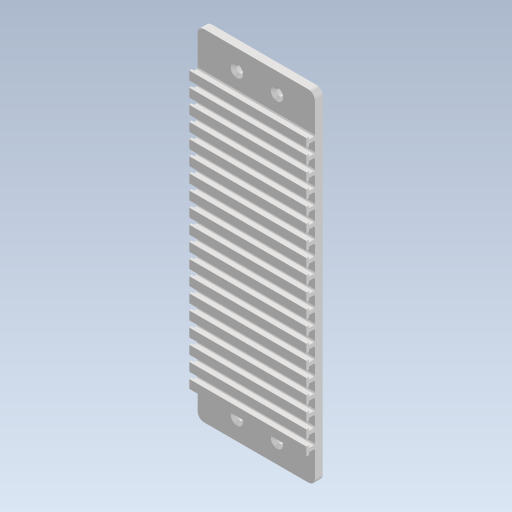
# Autodesk Inventor part: picadilly
Saved by Autodesk Inventor 2024 (Build 280153000, 153)
## iProperties
Created: 2024-06-10
Part Number: picadilly
Material: Типовые
Document SubType Name: Modeling
Designer: zhmis
Density: 1 g/cm^3
Appearance: По умолчанию
Author: zhmis
Autodesk Inventor part; units mm, degrees
ref_plane "YZ Plane" through (0, 0, 0) normal (1, 0, 0) x (0, 1, 0)
ref_plane "XZ Plane" through (0, 0, 0) normal (0, 1, 0) x (-1, 0, 0)
ref_plane "XY Plane" through (0, 0, 0) normal (0, 0, 1) x (1, 0, 0)
ref_plane "РабПлоскость1" through (0, 0, 0) normal (0, 0, 1) x (1, 0, 0)
sketch "Эскиз1" plane through (0, 0, 0) normal (0, 0, 1) x (1, 0, 0)
  circle A0 centre (-33.1299, -115.05) radius 1.65 projected
  circle A1 centre (-12.8537, -115.05) radius 1.65 projected
  circle A2 centre (-33.1299, 37.05) radius 1.65 projected
  circle A3 centre (-12.8537, 37.05) radius 1.65 projected
  line L0 (-52.9918, -117.55) -> (-52.9918, -99.275) projected
  line L1 (2.5082, -125.05) -> (-48.4918, -125.05) projected
  line L2 (2.5082, 47.05) -> (-48.4918, 47.05) projected
  line L3 (-52.9918, 39.55) -> (-52.9918, 21.275) projected
  line L4 (-52.9918, 43.875) -> (-52.9918, -121.875)
  line L5 (-49.8168, -125.05) -> (3.1042, -125.05)
  line L6 (6.2792, -121.875) -> (6.2792, 43.875)
  line L7 (3.1042, 47.05) -> (-49.8168, 47.05)
  arc A4 (-49.8168, 47.05) -> (-52.9918, 43.875) centre (-49.8168, 43.875) ccw
  arc A5 (6.2792, 43.875) -> (3.1042, 47.05) centre (3.1042, 43.875) ccw
  arc A6 (3.1042, -125.05) -> (6.2792, -121.875) centre (3.1042, -121.875) ccw
  arc A7 (-52.9918, -121.875) -> (-49.8168, -125.05) centre (-49.8168, -121.875) ccw
  point P0 (0, 0)
  point P1 (6.2792, 30.05)
  point P2 (-52.9918, 47.05)
  point P3 (-52.9918, -125.05)
  dimension "d0" = 3.175
  constraints: 8 end point, 8 point on circle, 8 tangent, 6 point on line, 4 centre point, 3 equal radius, 2 parallel, 1 perpendicular, 1 other
  measures "d0" radius of A4
extrude "Выдавливание1" add sketch "Эскиз1" along normal blind 4 contours A0 | A1 | A2 | A3 | L0 L4 L3 A4 L7 L2 A5 L6 A6 L5 L1 A7
sketch "Эскиз2" plane through (0, 0, 4) normal (0, 0, 1) x (1, 0, 0)
  circle A0 centre (-33.1299, -115.05) radius 1.65 projected
  circle A1 centre (-12.8537, -115.05) radius 1.65 projected
  circle A2 centre (-33.1299, 37.05) radius 1.65 projected
  circle A3 centre (-12.8537, 37.05) radius 1.65 projected
  point P0 (0, 0)
hole "Отверстие1" at (-12.8537, 37.05, 4) at (-33.1299, 37.05, 4) at (-12.8537, -115.05, 4) at (-33.1299, -115.05, 4) direction (0, 0, -1) diameter 3.4 depth 8.8 tip angle 118 countersink diameter 6.3 countersink angle 90 clearance for "Винт с потайной головкой ISO 2009/7046" size "M3" standard "ISO"
sketch "Эскиз4" plane through (-52.9918, -121.875, 0) normal (-1, 0, 0) x (0, 0, 1)
  line L0 (6.9999, 154.5045) -> (8.2499, 154.5045)
  line L1 (8.2499, 154.5045) -> (8.2499, 158.8045)
  line L2 (8.2499, 158.8045) -> (6.9999, 158.8045)
  line L3 (6.9999, 158.8045) -> (6.9999, 157.6045)
  line L4 (6.9999, 157.6045) -> (4.4999, 157.6045)
  line L5 (4.4999, 157.6045) -> (4.2499, 157.8545)
  line L6 (4.2499, 155.4545) -> (4.4999, 155.7045)
  line L7 (4.4999, 155.7045) -> (6.9999, 155.7045)
  line L8 (6.9999, 155.7045) -> (6.9999, 154.5045)
  line L9 (4.2499, 155.4545) -> (4, 155.2045)
  line L10 (4, 158.1044) -> (4.2499, 157.8545)
  line L11 (4, 158.1044) -> (4, 155.2045)
  line L12 (6.9999, 151.3045) -> (6.9999, 150.1045)
  line L13 (4.2499, 147.9545) -> (4, 147.7045)
  line L14 (4.4999, 150.1045) -> (4.2499, 150.3545)
  line L15 (4, 150.6044) -> (4.2499, 150.3545)
  line L16 (6.9999, 150.1045) -> (4.4999, 150.1045)
  line L17 (8.2499, 151.3045) -> (6.9999, 151.3045)
  line L18 (4.4999, 148.2045) -> (6.9999, 148.2045)
  line L19 (4.2499, 147.9545) -> (4.4999, 148.2045)
  line L20 (4, 150.6044) -> (4, 147.7045)
  line L21 (8.2499, 147.0045) -> (8.2499, 151.3045)
  line L22 (6.9999, 148.2045) -> (6.9999, 147.0045)
  line L23 (6.9999, 147.0045) -> (8.2499, 147.0045)
  line L24 (6.9999, 143.8045) -> (6.9999, 142.6045)
  line L25 (4.2499, 140.4545) -> (4, 140.2045)
  line L26 (4.4999, 142.6045) -> (4.2499, 142.8545)
  line L27 (4, 143.1044) -> (4.2499, 142.8545)
  line L28 (6.9999, 142.6045) -> (4.4999, 142.6045)
  line L29 (8.2499, 143.8045) -> (6.9999, 143.8045)
  line L30 (4.4999, 140.7045) -> (6.9999, 140.7045)
  line L31 (4.2499, 140.4545) -> (4.4999, 140.7045)
  line L32 (4, 143.1044) -> (4, 140.2045)
  line L33 (8.2499, 139.5045) -> (8.2499, 143.8045)
  line L34 (6.9999, 140.7045) -> (6.9999, 139.5045)
  line L35 (6.9999, 139.5045) -> (8.2499, 139.5045)
  line L36 (6.9999, 136.3045) -> (6.9999, 135.1045)
  line L37 (4.2499, 132.9545) -> (4, 132.7045)
  line L38 (4.4999, 135.1045) -> (4.2499, 135.3545)
  line L39 (4, 135.6044) -> (4.2499, 135.3545)
  line L40 (6.9999, 135.1045) -> (4.4999, 135.1045)
  line L41 (8.2499, 136.3045) -> (6.9999, 136.3045)
  line L42 (4.4999, 133.2045) -> (6.9999, 133.2045)
  line L43 (4.2499, 132.9545) -> (4.4999, 133.2045)
  line L44 (4, 135.6044) -> (4, 132.7045)
  line L45 (8.2499, 132.0045) -> (8.2499, 136.3045)
  line L46 (6.9999, 133.2045) -> (6.9999, 132.0045)
  line L47 (6.9999, 132.0045) -> (8.2499, 132.0045)
  line L48 (6.9999, 128.8045) -> (6.9999, 127.6045)
  line L49 (4.2499, 125.4545) -> (4, 125.2045)
  line L50 (4.4999, 127.6045) -> (4.2499, 127.8545)
  line L51 (4, 128.1044) -> (4.2499, 127.8545)
  line L52 (6.9999, 127.6045) -> (4.4999, 127.6045)
  line L53 (8.2499, 128.8045) -> (6.9999, 128.8045)
  line L54 (4.4999, 125.7045) -> (6.9999, 125.7045)
  line L55 (4.2499, 125.4545) -> (4.4999, 125.7045)
  line L56 (4, 128.1044) -> (4, 125.2045)
  line L57 (8.2499, 124.5045) -> (8.2499, 128.8045)
  line L58 (6.9999, 125.7045) -> (6.9999, 124.5045)
  line L59 (6.9999, 124.5045) -> (8.2499, 124.5045)
  line L60 (6.9999, 121.3045) -> (6.9999, 120.1045)
  line L61 (4.2499, 117.9545) -> (4, 117.7045)
  line L62 (4.4999, 120.1045) -> (4.2499, 120.3545)
  line L63 (4, 120.6044) -> (4.2499, 120.3545)
  line L64 (6.9999, 120.1045) -> (4.4999, 120.1045)
  line L65 (8.2499, 121.3045) -> (6.9999, 121.3045)
  line L66 (4.4999, 118.2045) -> (6.9999, 118.2045)
  line L67 (4.2499, 117.9545) -> (4.4999, 118.2045)
  line L68 (4, 120.6044) -> (4, 117.7045)
  line L69 (8.2499, 117.0045) -> (8.2499, 121.3045)
  line L70 (6.9999, 118.2045) -> (6.9999, 117.0045)
  line L71 (6.9999, 117.0045) -> (8.2499, 117.0045)
  line L72 (6.9999, 113.8045) -> (6.9999, 112.6045)
  line L73 (4.2499, 110.4545) -> (4, 110.2045)
  line L74 (4.4999, 112.6045) -> (4.2499, 112.8545)
  line L75 (4, 113.1044) -> (4.2499, 112.8545)
  line L76 (6.9999, 112.6045) -> (4.4999, 112.6045)
  line L77 (8.2499, 113.8045) -> (6.9999, 113.8045)
  line L78 (4.4999, 110.7045) -> (6.9999, 110.7045)
  line L79 (4.2499, 110.4545) -> (4.4999, 110.7045)
  line L80 (4, 113.1044) -> (4, 110.2045)
  line L81 (8.2499, 109.5045) -> (8.2499, 113.8045)
  line L82 (6.9999, 110.7045) -> (6.9999, 109.5045)
  line L83 (6.9999, 109.5045) -> (8.2499, 109.5045)
  line L84 (6.9999, 106.3045) -> (6.9999, 105.1045)
  line L85 (4.2499, 102.9545) -> (4, 102.7045)
  line L86 (4.4999, 105.1045) -> (4.2499, 105.3545)
  line L87 (4, 105.6044) -> (4.2499, 105.3545)
  line L88 (6.9999, 105.1045) -> (4.4999, 105.1045)
  line L89 (8.2499, 106.3045) -> (6.9999, 106.3045)
  line L90 (4.4999, 103.2045) -> (6.9999, 103.2045)
  line L91 (4.2499, 102.9545) -> (4.4999, 103.2045)
  line L92 (4, 105.6044) -> (4, 102.7045)
  line L93 (8.2499, 102.0045) -> (8.2499, 106.3045)
  line L94 (6.9999, 103.2045) -> (6.9999, 102.0045)
  line L95 (6.9999, 102.0045) -> (8.2499, 102.0045)
  line L96 (6.9999, 98.8045) -> (6.9999, 97.6045)
  line L97 (4.2499, 95.4545) -> (4, 95.2045)
  line L98 (4.4999, 97.6045) -> (4.2499, 97.8545)
  line L99 (4, 98.1044) -> (4.2499, 97.8545)
  line L100 (6.9999, 97.6045) -> (4.4999, 97.6045)
  line L101 (8.2499, 98.8045) -> (6.9999, 98.8045)
  line L102 (4.4999, 95.7045) -> (6.9999, 95.7045)
  line L103 (4.2499, 95.4545) -> (4.4999, 95.7045)
  line L104 (4, 98.1044) -> (4, 95.2045)
  line L105 (8.2499, 94.5045) -> (8.2499, 98.8045)
  line L106 (6.9999, 95.7045) -> (6.9999, 94.5045)
  line L107 (6.9999, 94.5045) -> (8.2499, 94.5045)
  line L108 (6.9999, 91.3045) -> (6.9999, 90.1045)
  line L109 (4.2499, 87.9545) -> (4, 87.7045)
  line L110 (4.4999, 90.1045) -> (4.2499, 90.3545)
  line L111 (4, 90.6044) -> (4.2499, 90.3545)
  line L112 (6.9999, 90.1045) -> (4.4999, 90.1045)
  line L113 (8.2499, 91.3045) -> (6.9999, 91.3045)
  line L114 (4.4999, 88.2045) -> (6.9999, 88.2045)
  line L115 (4.2499, 87.9545) -> (4.4999, 88.2045)
  line L116 (4, 90.6044) -> (4, 87.7045)
  line L117 (8.2499, 87.0045) -> (8.2499, 91.3045)
  line L118 (6.9999, 88.2045) -> (6.9999, 87.0045)
  line L119 (6.9999, 87.0045) -> (8.2499, 87.0045)
  line L120 (6.9999, 83.8045) -> (6.9999, 82.6045)
  line L121 (4.2499, 80.4545) -> (4, 80.2045)
  line L122 (4.4999, 82.6045) -> (4.2499, 82.8545)
  line L123 (4, 83.1044) -> (4.2499, 82.8545)
  line L124 (6.9999, 82.6045) -> (4.4999, 82.6045)
  line L125 (8.2499, 83.8045) -> (6.9999, 83.8045)
  line L126 (4.4999, 80.7045) -> (6.9999, 80.7045)
  line L127 (4.2499, 80.4545) -> (4.4999, 80.7045)
  line L128 (4, 83.1044) -> (4, 80.2045)
  line L129 (8.2499, 79.5045) -> (8.2499, 83.8045)
  line L130 (6.9999, 80.7045) -> (6.9999, 79.5045)
  line L131 (6.9999, 79.5045) -> (8.2499, 79.5045)
  line L132 (6.9999, 76.3045) -> (6.9999, 75.1045)
  line L133 (4.2499, 72.9545) -> (4, 72.7045)
  line L134 (4.4999, 75.1045) -> (4.2499, 75.3545)
  line L135 (4, 75.6044) -> (4.2499, 75.3545)
  line L136 (6.9999, 75.1045) -> (4.4999, 75.1045)
  line L137 (8.2499, 76.3045) -> (6.9999, 76.3045)
  line L138 (4.4999, 73.2045) -> (6.9999, 73.2045)
  line L139 (4.2499, 72.9545) -> (4.4999, 73.2045)
  line L140 (4, 75.6044) -> (4, 72.7045)
  line L141 (8.2499, 72.0045) -> (8.2499, 76.3045)
  line L142 (6.9999, 73.2045) -> (6.9999, 72.0045)
  line L143 (6.9999, 72.0045) -> (8.2499, 72.0045)
  line L144 (6.9999, 68.8045) -> (6.9999, 67.6045)
  line L145 (4.2499, 65.4545) -> (4, 65.2045)
  line L146 (4.4999, 67.6045) -> (4.2499, 67.8545)
  line L147 (4, 68.1044) -> (4.2499, 67.8545)
  line L148 (6.9999, 67.6045) -> (4.4999, 67.6045)
  line L149 (8.2499, 68.8045) -> (6.9999, 68.8045)
  line L150 (4.4999, 65.7045) -> (6.9999, 65.7045)
  line L151 (4.2499, 65.4545) -> (4.4999, 65.7045)
  line L152 (4, 68.1044) -> (4, 65.2045)
  line L153 (8.2499, 64.5045) -> (8.2499, 68.8045)
  line L154 (6.9999, 65.7045) -> (6.9999, 64.5045)
  line L155 (6.9999, 64.5045) -> (8.2499, 64.5045)
  line L156 (6.9999, 61.3045) -> (6.9999, 60.1045)
  line L157 (4.2499, 57.9545) -> (4, 57.7045)
  line L158 (4.4999, 60.1045) -> (4.2499, 60.3545)
  line L159 (4, 60.6044) -> (4.2499, 60.3545)
  line L160 (6.9999, 60.1045) -> (4.4999, 60.1045)
  line L161 (8.2499, 61.3045) -> (6.9999, 61.3045)
  line L162 (4.4999, 58.2045) -> (6.9999, 58.2045)
  line L163 (4.2499, 57.9545) -> (4.4999, 58.2045)
  line L164 (4, 60.6044) -> (4, 57.7045)
  line L165 (8.2499, 57.0045) -> (8.2499, 61.3045)
  line L166 (6.9999, 58.2045) -> (6.9999, 57.0045)
  line L167 (6.9999, 57.0045) -> (8.2499, 57.0045)
  line L168 (6.9999, 53.8045) -> (6.9999, 52.6045)
  line L169 (4.2499, 50.4545) -> (4, 50.2045)
  line L170 (4.4999, 52.6045) -> (4.2499, 52.8545)
  line L171 (4, 53.1044) -> (4.2499, 52.8545)
  line L172 (6.9999, 52.6045) -> (4.4999, 52.6045)
  line L173 (8.2499, 53.8045) -> (6.9999, 53.8045)
  line L174 (4.4999, 50.7045) -> (6.9999, 50.7045)
  line L175 (4.2499, 50.4545) -> (4.4999, 50.7045)
  line L176 (4, 53.1044) -> (4, 50.2045)
  line L177 (8.2499, 49.5045) -> (8.2499, 53.8045)
  line L178 (6.9999, 50.7045) -> (6.9999, 49.5045)
  line L179 (6.9999, 49.5045) -> (8.2499, 49.5045)
  line L180 (6.9999, 46.3045) -> (6.9999, 45.1045)
  line L181 (4.2499, 42.9545) -> (4, 42.7045)
  line L182 (4.4999, 45.1045) -> (4.2499, 45.3545)
  line L183 (4, 45.6044) -> (4.2499, 45.3545)
  line L184 (6.9999, 45.1045) -> (4.4999, 45.1045)
  line L185 (8.2499, 46.3045) -> (6.9999, 46.3045)
  line L186 (4.4999, 43.2045) -> (6.9999, 43.2045)
  line L187 (4.2499, 42.9545) -> (4.4999, 43.2045)
  line L188 (4, 45.6044) -> (4, 42.7045)
  line L189 (8.2499, 42.0045) -> (8.2499, 46.3045)
  line L190 (6.9999, 43.2045) -> (6.9999, 42.0045)
  line L191 (6.9999, 42.0045) -> (8.2499, 42.0045)
  line L192 (6.9999, 38.8045) -> (6.9999, 37.6045)
  line L193 (4.2499, 35.4545) -> (4, 35.2045)
  line L194 (4.4999, 37.6045) -> (4.2499, 37.8545)
  line L195 (4, 38.1044) -> (4.2499, 37.8545)
  line L196 (6.9999, 37.6045) -> (4.4999, 37.6045)
  line L197 (8.2499, 38.8045) -> (6.9999, 38.8045)
  line L198 (4.4999, 35.7045) -> (6.9999, 35.7045)
  line L199 (4.2499, 35.4545) -> (4.4999, 35.7045)
  line L200 (4, 38.1044) -> (4, 35.2045)
  line L201 (8.2499, 34.5045) -> (8.2499, 38.8045)
  line L202 (6.9999, 35.7045) -> (6.9999, 34.5045)
  line L203 (6.9999, 34.5045) -> (8.2499, 34.5045)
  line L204 (6.9999, 31.3045) -> (6.9999, 30.1045)
  line L205 (4.2499, 27.9545) -> (4, 27.7045)
  line L206 (4.4999, 30.1045) -> (4.2499, 30.3545)
  line L207 (4, 30.6044) -> (4.2499, 30.3545)
  line L208 (6.9999, 30.1045) -> (4.4999, 30.1045)
  line L209 (8.2499, 31.3045) -> (6.9999, 31.3045)
  line L210 (4.4999, 28.2045) -> (6.9999, 28.2045)
  line L211 (4.2499, 27.9545) -> (4.4999, 28.2045)
  line L212 (4, 30.6044) -> (4, 27.7045)
  line L213 (8.2499, 27.0045) -> (8.2499, 31.3045)
  line L214 (6.9999, 28.2045) -> (6.9999, 27.0045)
  line L215 (6.9999, 27.0045) -> (8.2499, 27.0045)
  line L216 (6.9999, 23.8045) -> (6.9999, 22.6045)
  line L217 (4.2499, 20.4545) -> (4, 20.2045)
  line L218 (4.4999, 22.6045) -> (4.2499, 22.8545)
  line L219 (4, 23.1044) -> (4.2499, 22.8545)
  line L220 (6.9999, 22.6045) -> (4.4999, 22.6045)
  line L221 (8.2499, 23.8045) -> (6.9999, 23.8045)
  line L222 (4.4999, 20.7045) -> (6.9999, 20.7045)
  line L223 (4.2499, 20.4545) -> (4.4999, 20.7045)
  line L224 (4, 23.1044) -> (4, 20.2045)
  line L225 (8.2499, 19.5045) -> (8.2499, 23.8045)
  line L226 (6.9999, 20.7045) -> (6.9999, 19.5045)
  line L227 (6.9999, 19.5045) -> (8.2499, 19.5045)
  line L228 (6.9999, 16.3045) -> (6.9999, 15.1045)
  line L229 (4.2499, 12.9545) -> (4, 12.7045)
  line L230 (4.4999, 15.1045) -> (4.2499, 15.3545)
  line L231 (4, 15.6044) -> (4.2499, 15.3545)
  line L232 (6.9999, 15.1045) -> (4.4999, 15.1045)
  line L233 (8.2499, 16.3045) -> (6.9999, 16.3045)
  line L234 (4.4999, 13.2045) -> (6.9999, 13.2045)
  line L235 (4.2499, 12.9545) -> (4.4999, 13.2045)
  line L236 (4, 15.6044) -> (4, 12.7045)
  line L237 (8.2499, 12.0045) -> (8.2499, 16.3045)
  line L238 (6.9999, 13.2045) -> (6.9999, 12.0045)
  line L239 (6.9999, 12.0045) -> (8.2499, 12.0045)
  dimension "d21" = 7.5
  constraints: 480 end point, 1 collinear, 1 vertical, 455 other
  measures "d21" distance of L2.end L12.start
extrude "Выдавливание2" add sketch "Эскиз4" against normal up to surface (59.271 mm away) contours L17 L21 L23 L22 L18 L19 L13 L20 L15 L14 L16 L12 | L29 L33 L35 L34 L30 L31 L25 L32 L27 L26 L28 L24 | L41 L45 L47 L46 L42 L43 L37 L44 L39 L38 L40 L36 | L53 L57 L59 L58 L54 L55 L49 L56 L51 L50 L52 L48 | L65 L69 L71 L70 L66 L67 L61 L68 L63 L62 L64 L60 | L77 L81 L83 L82 L78 L79 L73 L80 L75 L74 L76 L72 | L89 L93 L95 L94 L90 L91 L85 L92 L87 L86 L88 L84 | L101 L105 L107 L106 L102 L103 L97 L104 L99 L98 L100 L96 | L113 L117 L119 L118 L114 L115 L109 L116 L111 L110 L112 L108 | L125 L129 L131 L130 L126 L127 L121 L128 L123 L122 L124 L120 | L137 L141 L143 L142 L138 L139 L133 L140 L135 L134 L136 L132 | L149 L153 L155 L154 L150 L151 L145 L152 L147 L146 L148 L144 | L161 L165 L167 L166 L162 L163 L157 L164 L159 L158 L160 L156 | L173 L177 L179 L178 L174 L175 L169 L176 L171 L170 L172 L168 | L185 L189 L191 L190 L186 L187 L181 L188 L183 L182 L184 L180 | L197 L201 L203 L202 L198 L199 L193 L200 L195 L194 L196 L192 | L209 L213 L215 L214 L210 L211 L205 L212 L207 L206 L208 L204 | L221 L225 L227 L226 L222 L223 L217 L224 L219 L218 L220 L216 | L233 L237 L239 L238 L234 L235 L229 L236 L231 L230 L232 L228
